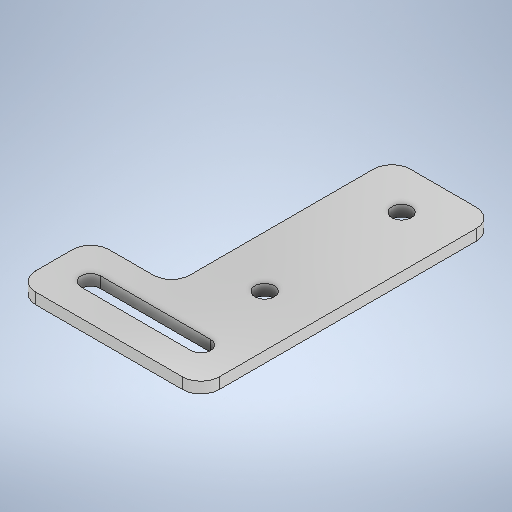
# Autodesk Inventor part: LeadScrewEndMount
Saved by Autodesk Inventor 2025.2 (Build 292293000, 293)
## iProperties
Created: 2025-07-28
Part Number: LeadScrewEndMount
Material: Generic
Document SubType Name: Modeling
Designer: Simon
Density: 1 g/cm^3
Appearance: Aluminum - Dark
Author: Simon
Autodesk Inventor part; units mm, degrees
ref_plane "YZ Plane" through (0, 0, 0) normal (1, 0, 0) x (0, 1, 0)
ref_plane "XZ Plane" through (0, 0, 0) normal (0, 1, 0) x (-1, 0, 0)
ref_plane "XY Plane" through (0, 0, 0) normal (0, 0, 1) x (1, 0, 0)
sketch "Sketch1" plane through (0, 0, 0) normal (0, 1, 0) x (-1, 0, 0)
  line L0 (-25, 40) -> (25, 40)
  line L1 (25, 40) -> (25, -40)
  line L2 (25, -40) -> (-25, -40)
  line L3 (-25, -40) -> (-25, 40)
  line L4 (-25, 40) -> (25, -40) construction
  line L5 (25, 40) -> (-25, -40) construction
  point P0 (0, 0)
  dimension "d0" = 50
  dimension "d1" = 80
  constraints: 12 end point, 2 midpoint, 2 parallel, 1 horizontal, 1 perpendicular
  measures "d0" distance of L1.end L2.end
  measures "d1" distance of L0.end L1.end
extrude "Extrusion1" add sketch "Sketch1" along normal blind 3
sketch "Sketch2" plane through (0, 3, 0) normal (0, 1, 0) x (1, 0, 0)
  line L0 (25, -40) -> (25, 40) projected
  line L1 (25, 40) -> (11, 40)
  line L2 (11, 40) -> (11, 28.65)
  line L3 (11, 28.65) -> (25, 28.65)
  line L4 (25, 28.65) -> (25, 40)
  line L5 (11, 28.65) -> (11, -8.65)
  circle A0 centre (11, 28.65) radius 2.65
  circle A1 centre (11, -8.65) radius 2.65
  line L6 (-25, -40) -> (25, -40) projected
  line L7 (-25, 40) -> (-25, -40) projected
  line L8 (25, -40) -> (-25, -40)
  line L9 (-25, -40) -> (-25, -30)
  line L10 (-25, -30) -> (25, -30)
  line L11 (25, -30) -> (25, -40)
  line L12 (25, -30) -> (15, -30)
  line L13 (-25, -30) -> (-15, -30)
  line L14 (-15, -30) -> (15, -30) construction
  line L15 (-15, -32.65) -> (15, -32.65)
  line L16 (15, -27.35) -> (-15, -27.35)
  arc A2 (-15, -27.35) -> (-15, -32.65) centre (-15, -30) ccw
  arc A3 (15, -32.65) -> (15, -27.35) centre (15, -30) ccw
  line L17 (-25, -30) -> (-25, 40)
  line L18 (-25, 40) -> (-3, 40)
  line L19 (-3, 40) -> (-3, -20)
  line L20 (-3, -20) -> (-25, -20)
  point P0 (0, 0)
  point P1 (0, -30)
  dimension "d4" = 14
  dimension "d5" = 11.35
  dimension "d6" = 37.3
  dimension "d7" = 5.3
  dimension "d8" = 5.3
  dimension "d9" = 10
  dimension "d10" = 10
  dimension "d11" = 10
  dimension "d12" = 5.3
  dimension "d13" = 22
  dimension "d14" = 60
  constraints: 38 end point, 5 parallel, 5 perpendicular, 4 centre point, 4 point on circle, 4 point on line, 4 tangent, 2 coincident, 2 collinear, 2 horizontal, 1 midpoint, 1 vertical
  measures "d4" distance of L3.end L2.end
  measures "d5" distance of L2.end L1.end
  measures "d6" distance of L2.end L5.end
  measures "d7" diameter of A0
  measures "d8" diameter of A1
  measures "d9" distance of L8.end L9.end
  measures "d10" distance of L10.end L12.end
  measures "d11" distance of L9.end L13.end
  measures "d12" diameter of A3
  measures "d13" distance of L7.start L18.end
  measures "d14" distance of L18.end L19.end
extrude "Extrusion2" cut sketch "Sketch2" against normal through all contours L7 L18 L19 L20 | A1 | A3 L15 A2 L10 | L10 A2 L16 A3 | A0 L5 L3 | L3 L2 A0 | L5 A0 L2
fillet "Fillet1" radius 5 6 edges at (-25, 1.5, 40) (25, 1.5, 40) (25, 1.5, -40) (-3, 1.5, -40) (-3, 1.5, 20) (-25, 1.5, 20)
body "Solid1"
